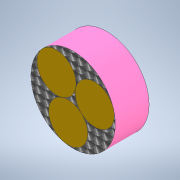
# Autodesk Inventor part: LED and carclo
Saved by Autodesk Inventor 2021 (Build 250183000, 183)
## iProperties
Created: 2020-10-20
Part Number: LED and carclo
Material: Generic
Document SubType Name: Modeling
Designer: VM
Density: 1 g/cm^3
Appearance: Default
Author: VM
Autodesk Inventor part; units mm, degrees
ref_plane "YZ Plane" through (0, 0, 0) normal (1, 0, 0) x (0, 1, 0)
ref_plane "XZ Plane" through (0, 0, 0) normal (0, 1, 0) x (-1, 0, 0)
ref_plane "XY Plane" through (0, 0, 0) normal (0, 0, 1) x (1, 0, 0)
sketch "Sketch1" plane through (0, 0, 0) normal (0, 0, 1) x (1, 0, 0)
  circle A0 centre (0, 0) radius 10
  dimension "d0" = 20
  constraints: 1 centre point, 1 coincident
  measures "d0" diameter of A0
extrude "Extrusion1" add sketch "Sketch1" along normal blind 8
sketch "Sketch2" plane through (0, 0, 8) normal (0, 0, 1) x (1, 0, 0)
  circle A0 centre (-3.9419, 3.6305) radius 4.641
  circle A1 centre (5.115, 1.5985) radius 4.641
  circle A2 centre (-1.1732, -5.229) radius 4.641
  circle A3 centre (0, 0) radius 10 projected
  circle A4 centre (0, 0) radius 10 projected
  point P0 (1.9709, -1.8152)
  point P1 (-2.5575, -0.7993)
  point P2 (0.5866, 2.6145)
  constraints: 6 tangent, 3 centre point, 2 equal radius
extrude "Extrusion2" cut sketch "Sketch2" against normal blind 0.01 contours A0 | A1 | A2
body "Solid1"
